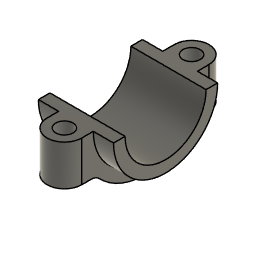
Rod Cap_ (Autodesk Fusion 360 design; units mm, degrees)
Autodesk Fusion 360 part; units mm, degrees
note: some values were not read from the file. Chosen so that the rebuilt part matches the saved one: which face or edge a step refers to; which pieces of a blend or face edit are solid.
sketch "Sketch1" plane through (0, 0, 0) normal (1, 0, 0) x (0, 1, 0)
  arc A0 (-177.8, 0) -> (177.8, 0) centre (0, 0) ccw
  arc A1 (-228.6, 0) -> (228.6, 0) centre (0, 0) ccw
  line L0 (-228.6, 0) -> (-177.8, 0)
  line L1 (177.8, 0) -> (228.6, 0)
  dimension "d1" = 177.8
  dimension "d2" = 50.8
  constraint coincident A0.centre A1.centre
  constraint horizontal A0.centre A0.start
  constraint horizontal A0.centre A0.end
  constraint horizontal L0
  constraint parallel L0 L1
  measures "d1" radius of A0
extrude "Extrude1" add sketch "Sketch1" along normal mid plane 330.2
sketch "Sketch2" plane through (0, 0, 0) normal (1, 0, 0) x (0, 1, 0)
  arc A0 (-279.4, 0) -> (279.4, 0) centre (0, 0) ccw
  line L0 (0, 0) -> (0, -516.6441) construction
  arc A1 (-228.6, 0) -> (228.6, 0) centre (0, 0) ccw
  line L1 (-228.6, 0) -> (-355.6, 0)
  line L2 (-355.6, 0) -> (-355.6, -177.8)
  line L3 (-355.6, -177.8) -> (-215.5261, -177.8)
  line L4 (355.6, 0) -> (355.6, -177.8)
  line L5 (355.6, -177.8) -> (215.5261, -177.8)
  line L6 (228.6, 0) -> (355.6, 0)
  dimension "d5" = 279.4
  dimension "d6" = 355.6
  dimension "d7" = 177.8
  constraint coincident A0.centre L0.start
  constraint vertical L0
  constraint coincident A1.start L1.start
  constraint horizontal L1
  constraint perpendicular L1 L2
  constraint coincident A0 L3.end
  constraint perpendicular L2 L3
  constraint symmetric L0 A1.start A1.end
  constraint symmetric L0 L1.end L4.start
  constraint symmetric L0 L2.end L4.end
  constraint symmetric L0 L3.end L5.end
  measures "d5" radius of A0
  measures "d6" distance of A0.centre L2
  measures "d7" distance of L1.end L2.end
extrude "Extrude2" add sketch "Sketch2" along normal mid plane 152.4
fillet "Fillet1" radius 25.4 2 edges at (76.2, -285.5631, -177.8) (76.2, 0, -228.6)
fillet "Fillet1" radius 76.2 2 edges at (-76.2, 355.6, -88.9) (76.2, 355.6, -88.9)
fillet "Fillet1" radius 25.4 2 edges at (-76.2, -285.5631, -177.8) (-76.2, 0, -228.6)
fillet "Fillet1" radius 76.2 2 edges at (-76.2, -355.6, -88.9) (76.2, -355.6, -88.9)
sketch "Sketch3" plane through (0, 0, 0) normal (0, 0, 1) x (-1, 0, 0)
  arc A0 (76.2, 279.4) -> (-76.2, 279.4) centre (0, 279.4) ccw
  line L0 (-76.2, 279.4) -> (-76.2, 228.6)
  line L1 (-76.2, 228.6) -> (-165.1, 228.6)
  line L2 (-165.1, 228.6) -> (-165.1, 177.8)
  line L3 (-165.1, 177.8) -> (165.1, 177.8)
  line L4 (165.1, 177.8) -> (165.1, 228.6)
  line L5 (165.1, 228.6) -> (76.2, 228.6)
  line L6 (76.2, 228.6) -> (76.2, 279.4)
  circle A1 centre (0, 279.4) radius 38.1
  circle A2 centre (0, -279.4) radius 38.1
  arc A3 (-76.2, -279.4) -> (76.2, -279.4) centre (0, -279.4) ccw
  dimension "d10" = 76.2
  dimension "d11" = 76.2
  constraint concentric A0 A1
  constraint concentric A2 A3
  measures "d10" diameter of A1
  measures "d11" diameter of A2
extrude "Extrude3" cut sketch "Sketch3" against normal blind 228.6 contours A1 | A2
fillet "Fillet2" radius 50.8 2 edges at (0, -215.5261, -177.8) (0, 215.5261, -177.8)
